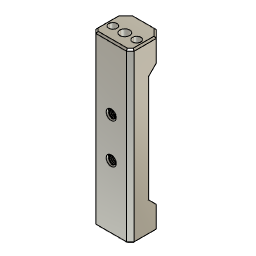
Apollo Yoke Lamp Mount Body [(M)SPPS000000036] v2 (Autodesk Fusion 360 design; units mm, degrees)
Autodesk Fusion 360 part; units mm, degrees
sketch "Sketch1" plane through (0, 0, 0) normal (1, 0, 0) x (0, 1, 0)
  line L0 (-12, -55) -> (10, -55)
  line L1 (10, -55) -> (10, 55)
  line L2 (10, 55) -> (-12, 55)
  line L3 (-12, 55) -> (-12, -55)
  line L4 (0, 55) -> (0, -55)
  line L5 (10, 35) -> (-12, 35)
  line L6 (-12, -35) -> (10, -35)
  dimension "d158" = 22
  dimension "d5" = 110
  dimension "d6" = 12
  dimension "d7" = 55
  dimension "d8" = 20
  dimension "d9" = 20
  dimension "d10" = 12
  constraint horizontal L2
  constraint vertical L3
  constraint horizontal L0
  constraint vertical L1
  constraint parallel L3 L4
  constraint coincident L2 L4.start
  constraint coincident L0 L4.end
  constraint parallel L2 L5
  constraint coincident L3 L5.end
  constraint coincident L1 L5.start
  constraint coincident L1 L6.end
  constraint coincident L3 L6.start
  measures "d158" distance of L1 L3
  measures "d5" distance of L0 L2
  measures "d6" distance of L3 L4
  measures "d7" distance of origin L2
  measures "d8" distance of L2 L5
  measures "d9" distance of L0 L6
  measures "d10" distance of origin L3
extrude "Extrude1" add sketch "Sketch1" along normal mid plane 25 contours L0 L3 L4 L6 | L0 L1 L4 L6 | L3 L4 L5 L6 | L2 L3 L4 L5 | L1 L2 L4 L5
chamfer "Chamfer1" distance 10 angle 45 2 edges at (0, 10, 35) (0, 10, -35)
sketch "Sketch2" plane through (0, 0, -55) normal (0, 0, -1) x (1, 0, 0)
  line L0 (-12.5, -10) -> (12.5, -10)
  line L1 (12.5, -10) -> (12.5, 12)
  line L2 (12.5, 12) -> (-12.5, 12)
  line L3 (-12.5, 12) -> (-12.5, -10)
  circle A0 centre (7.8, 3.1) radius 2.2
  circle A1 centre (7.8, 3.1) radius 2.7
  circle A2 centre (0, 3.1) radius 3.2
  circle A3 centre (-7.8, 3.1) radius 2.7
  circle A4 centre (-7.8, 3.1) radius 2.2
  line L4 (-4, 6.6) -> (4, 6.6)
  line L5 (4, 6.6) -> (4, -10)
  line L6 (4, -10) -> (-4, -10)
  line L7 (-4, -10) -> (-4, 6.6)
  dimension "d162" = 6.4
  dimension "d223" = 5.4
  dimension "d224" = 5.4
  dimension "d225" = 4.4
  dimension "d226" = 4.4
  dimension "d227" = 15.6
  dimension "d20" = 8.9
  dimension "d21" = 7.8
  dimension "d34" = 8
  dimension "d35" = 4
  dimension "d36" = 5.4
  constraint concentric A0 A1
  constraint concentric A3 A4
  constraint horizontal A0.centre A2.centre
  constraint horizontal A3.centre A2.centre
  constraint vertical origin A2.centre
  constraint horizontal L4
  constraint vertical L5
  constraint horizontal L6
  constraint vertical L7
  constraint coincident L0 L5.end
  measures "d162" diameter of A2
  measures "d223" diameter of A1
  measures "d224" diameter of A3
  measures "d225" diameter of A0
  measures "d226" diameter of A4
  measures "d227" distance of A3.centre A0.centre
  measures "d20" distance of L2 A0.centre
  measures "d21" horizontal distance of origin A0.centre
  measures "d34" distance of L5 L7
  measures "d35" distance of A2.centre L5
  measures "d36" distance of L2 L4
extrude "Extrude2" cut sketch "Sketch2" against normal blind 111 contours A2
sketch "Sketch3" plane through (0, -12, 0) normal (0, -1, 0) x (1, 0, 0)
  line L0 (-12.5, -55) -> (12.5, -55)
  line L1 (12.5, -55) -> (12.5, 55)
  line L2 (12.5, 55) -> (-12.5, 55)
  line L3 (-12.5, 55) -> (-12.5, -55)
  circle A0 centre (0, 13) radius 3.2
  circle A1 centre (0, 0) radius 2
  circle A2 centre (0, -13) radius 3.2
  dimension "d169" = 4
  dimension "d170" = 6.4
  dimension "d171" = 6.4
  dimension "d172" = 26
  dimension "d173" = 13
  constraint coincident A1.centre origin
  constraint vertical A1.centre A0.centre
  constraint vertical A1.centre A2.centre
  measures "d169" diameter of A1
  measures "d170" diameter of A2
  measures "d171" diameter of A0
  measures "d172" distance of A2.centre A0.centre
  measures "d173" distance of A1.centre A0.centre
hole "Hole1" at (0, -12, -13) at (0, -12, 13) direction (0, 1, 0) diameter 5.035 depth 9 tip angle 118 countersink diameter 6.6 countersink angle 90
thread "Thread1" "ISO Metric profile 6.0 M6x1 6H" major diameter 6.147 minor diameter 5.035 pitch 1 angle 60 modelled right hand crest width 0.2748 on face at (2.5175, -9.1701, -12.9963) crest through (0, -10.9675, -15.5175) on face at (2.5175, -9.1701, 13.0037) crest through (0, -10.9675, 10.4825)
extrude "Extrude3" cut sketch "Sketch2" against normal blind 80 from surface at -15 contours L0 L4 L5 L6 L7
fillet "Fillet1" radius 4 4 edges at (-4, -0.8, 40) (4, -0.8, 40) (-4, -0.8, -40) (4, -0.8, -40)
chamfer "Chamfer2" distance 5 angle 45 4 edges at (-12.5, 10, 50) (12.5, 10, 50) (-12.5, 10, -50) (12.5, 10, -50)
chamfer "Chamfer3" distance 2.5 angle 45 2 edges at (12.5, -12, 0) (-12.5, -12, 0)
chamfer "Chamfer4" distance 1 angle 45 16 edges at (0, 10, 55) (10, 7.5, 55) (12.5, -2.25, 55) (11.25, -10.75, 55) (0, -12, 55) (-11.25, -10.75, 55) (-12.5, -2.25, 55) (-10, 7.5, 55) (0, 10, -55) (10, 7.5, -55) (12.5, -2.25, -55) (11.25, -10.75, -55) (0, -12, -55) (-10, 7.5, -55) (-12.5, -2.25, -55) (-11.25, -10.75, -55)
extrude "Extrude4" cut sketch "Sketch2" against normal blind 14 contours A0 | A1 | A3 | A4
extrude "Extrude5" cut sketch "Sketch2" along normal blind 14 from surface at -110 contours A0 | A1 | A3 | A4
equation "d7 = d5 / 2"
equation "d21 = d227 / 2"
equation "d173 = d172 / 2"
equation "d35 = d34 / 2"
